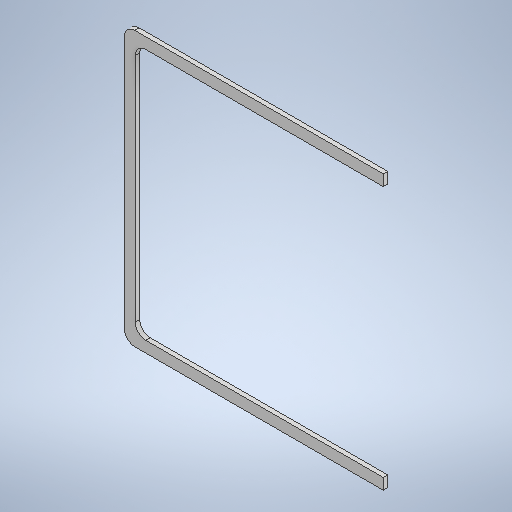
# Autodesk Inventor part: Опоры на кожухе
Saved by Autodesk Inventor 2025 (Build 290162010, 162A)
## iProperties
Created: 2024-07-07
Part Number: Опоры на кожухе
Material: Stainless Steel
Document SubType Name: Sheet Metal
Designer: pokla
Density: 8 g/cm^3
Sheet Metal Rule: AISI304 2mm Die16
Appearance: Default
Author: pokla
Autodesk Inventor part; units mm, degrees
ref_plane "YZ Plane" through (0, 0, 0) normal (1, 0, 0) x (0, 1, 0)
ref_plane "XZ Plane" through (0, 0, 0) normal (0, 1, 0) x (-1, 0, 0)
ref_plane "XY Plane" through (0, 0, 0) normal (0, 0, 1) x (1, 0, 0)
sketch "Sketch1" plane through (0, 0, 0) normal (0, 1, 0) x (-1, 0, 0)
  line L0 (0, 62) -> (0, 57.25) construction
  line L1 (0, 62) -> (-4.75, 62) construction
  line L2 (0, -62) -> (-4.75, -62) construction
  line L3 (-117.25, -57) -> (-9.75, -57)
  line L4 (-5, -57) -> (-5, -52.25) construction
  line L5 (-5, 57) -> (-9.75, 57) construction
  line L6 (-117.25, 57) -> (-117.25, 62)
  line L7 (-117.25, -62) -> (-117.25, -57)
  arc A0 (-5, 52.25) -> (-9.75, 57) centre (-9.75, 52.25) ccw
  arc A1 (-9.75, -57) -> (-5, -52.25) centre (-9.75, -52.25) ccw
  arc A2 (0, 57.25) -> (-4.75, 62) centre (-4.75, 57.25) ccw
  arc A3 (-4.75, -62) -> (0, -57.25) centre (-4.75, -57.25) ccw
  line L8 (0, 57.25) -> (0, -57.25)
  line L9 (-4.75, 62) -> (-117.25, 62)
  line L10 (0, -57.25) -> (0, -62) construction
  line L11 (-4.75, -62) -> (-117.25, -62)
  line L12 (-5, -52.25) -> (-5, 52.25)
  line L13 (-9.75, -57) -> (-5, -57) construction
  line L14 (-5, 52.25) -> (-5, 57) construction
  line L15 (-9.75, 57) -> (-117.25, 57)
  arc A4 (-4.75, 62) -> (0, 57.25) centre (-4.75, 57.25) ccw construction
  arc A5 (-9.75, 57) -> (-5, 52.25) centre (-9.75, 52.25) ccw construction
  arc A6 (0, -57.25) -> (-4.75, -62) centre (-4.75, -57.25) ccw construction
  arc A7 (-5, -52.25) -> (-9.75, -57) centre (-9.75, -52.25) ccw construction
  point P0 (0, 0)
  point P1 (0, 0)
  dimension "d4" = 5
  dimension "d6" = 117.25
  dimension "d8" = 117.25
  dimension "d9" = 5
  dimension "d10" = 5
  dimension "d11" = 124
  dimension "d12" = 57
  dimension "d14" = 9.5
  measures "d4" distance between parallel lines of L0 L4
  measures "d6" distance between parallel lines of L6 L0
  measures "d8" distance from line of point (0, 0) L7
  measures "d9" distance of L6.start L6.end
  measures "d10" distance of L7.start L3.start
  measures "d11" distance of L0.start L2.start
  measures "d12" distance from line of point (0, 0) L3
  measures "d14" diameter of A2
extrude "Plate1" add sketch "Sketch1" against normal blind 2
equation "\"d8\" = d6"
equation "\"d9\" = d4"
equation "\"d10\" = d4"
equation "\"d11\" = Ширина_крепления_корпуса + 2 * Thickness"
equation "\"d5\" = Thickness"
equation "\"BendReliefWidth\" = Thickness"
equation "\"BendReliefDepth\" = 0.5 * Thickness"
equation "\"CornerReliefSize\" = 4 * Thickness"
equation "\"MinimumRemnant\" = 2 * Thickness"
equation "\"TransitionRadius\" = BendRadius"
equation "\"JacobiRadiusSize\" = BendRadius"
equation "\"GapSize\" = Thickness"
equation "\"Ширина_крепления_корпуса\" = 120"
equation "\"Thickness\" = 2"
equation "\"BendRadius\" = 2.75"
body "Solid1"
